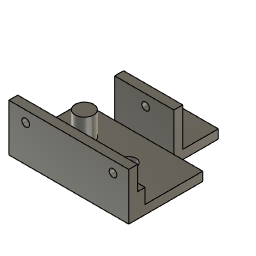
RoboCrab Top v3 (Autodesk Fusion 360 design; units mm, degrees)
Autodesk Fusion 360 part; units mm, degrees
sketch "Base" plane through (0, 0, 0) normal (0, 0, 1) x (1, 0, 0)
  line L0 (-9.4551, 20.4231) -> (10.5449, 20.4231)
  line L1 (20.2949, 5.4231) -> (20.2949, -19.5769)
  line L2 (20.2949, -19.5769) -> (-20.2051, -19.5769)
  line L3 (-20.2051, -19.5769) -> (-20.2051, 5.4231)
  line L4 (-20.2051, 5.4231) -> (-9.4551, 5.4231)
  line L5 (-9.4551, 5.4231) -> (-9.4551, 20.4231)
  line L6 (10.5449, 20.4231) -> (10.5449, 5.4231)
  line L7 (10.5449, 5.4231) -> (20.2949, 5.4231)
  dimension "d1" = 40
  dimension "d2" = 40.5
  dimension "d3" = 25
  dimension "d4" = 25
  dimension "d5" = 10.75
  dimension "d6" = 20
  constraint horizontal L0
  constraint vertical L1
  constraint horizontal L2
  constraint vertical L3
  constraint perpendicular L3 L4
  constraint perpendicular L0 L5
  constraint perpendicular L0 L6
  constraint perpendicular L1 L7
  measures "d1" distance of L0 L2
  measures "d2" distance of L1 L3
  measures "d3" distance of L2 L4
  measures "d4" distance of L2 L7
  measures "d5" distance of L3.end L4.end
  measures "d6" distance of L5 L6
extrude "Extrude1" add sketch "Base" along normal blind 3
sketch "Messurements" plane through (0, 0, 3) normal (0, 0, 1) x (-1, 0, 0)
  line L0 (-10.5449, -5.4231) -> (-10.5449, -20.4231)
  line L1 (-10.5449, -20.4231) -> (9.4551, -20.4231)
  line L2 (9.4551, -20.4231) -> (9.4551, -5.4231)
  line L3 (9.4551, -5.4231) -> (20.2051, -5.4231)
  line L4 (20.2051, -5.4231) -> (20.2051, 19.5769)
  line L5 (20.2051, 19.5769) -> (-20.2949, 19.5769)
  line L6 (-20.2949, 19.5769) -> (-20.2949, -5.4231)
  line L7 (-20.2949, -5.4231) -> (-10.5449, -5.4231)
  line L8 (20.2051, 14.0769) -> (-20.2949, 14.0769)
  line L9 (9.4551, -5.4231) -> (-10.5449, -5.4231)
  line L10 (9.4551, -8.4231) -> (-10.5449, -8.4231)
  circle A0 centre (-5.2949, 4.5769) radius 2.5
  circle A1 centre (9.6801, 4.5769) radius 3.125
  dimension "d9" = 5.5
  dimension "d10" = 3
  dimension "d11" = 5
  dimension "d12" = 6.25
  dimension "d13" = 15
  dimension "d14" = 10
  dimension "d15" = 10
  dimension "d16" = 10.525
  constraint coincident L4 L8.start
  constraint coincident L6 L8.end
  constraint perpendicular L6 L8
  constraint coincident L2.end L3.start
  constraint coincident L0.start L7.end
  constraint coincident L2 L10.start
  constraint coincident L0 L10.end
  constraint perpendicular L0 L10
  measures "d9" distance of L5 L8
  measures "d10" distance of L9 L10
  measures "d11" diameter of A0
  measures "d12" diameter of A1
  measures "d13" distance of L6 A0.centre
  measures "d14" distance of L9 A0.centre
  measures "d15" distance of L9 A1.centre
  measures "d16" distance of L4 A1.centre
extrude "Extrude2" cut sketch "Messurements" against normal blind 2 contours A0
extrude "Extrude3" add sketch "Messurements" along normal blind 8 contours A1
extrude "Extrude4" add sketch "Messurements" along normal blind 5 contours L4 L5 L6 L8
extrude "Extrude5" add sketch "Messurements" along normal blind 13 contours L0 L2 L9 L10
sketch "Other" plane through (0, 0, 8) normal (0, 0, 1) x (-1, 0, 0)
  line L0 (20.2051, 19.5769) -> (-20.2949, 19.5769)
  line L1 (-20.2949, 19.5769) -> (-20.2949, 14.0769)
  line L2 (-20.2949, 14.0769) -> (20.2051, 14.0769)
  line L3 (20.2051, 14.0769) -> (20.2051, 19.5769)
  line L4 (20.2051, 14.0769) -> (-20.2949, 14.0769)
  line L5 (-20.2949, 16.5769) -> (20.2051, 16.5769)
  dimension "d28" = 2.5
  constraint coincident L1 L5.start
  constraint coincident L3 L5.end
  constraint perpendicular L3 L5
  measures "d28" distance of L4 L5
extrude "Extrude6" add sketch "Other" along normal blind 8 contours L0 L1 L3 L5
sketch "Attachment2" plane through (0, -16.5769, 0) normal (0, 1, 0) x (-1, 0, 0)
  line L0 (-20.2949, 8) -> (20.2051, 8)
  line L1 (20.2051, 8) -> (20.2051, 16)
  line L2 (20.2051, 16) -> (-20.2949, 16)
  line L3 (-20.2949, 16) -> (-20.2949, 8)
  circle A0 centre (-14.9949, 12.3) radius 1.3
  circle A1 centre (14.5051, 12.3) radius 1.3
  dimension "d31" = 2.6
  dimension "d32" = 3.7
  dimension "d33" = 5.3
  dimension "d34" = 2.6
  dimension "d35" = 5.7
  dimension "d36" = 3.7
  measures "d31" diameter of A0
  measures "d32" distance of L2 A0.centre
  measures "d33" distance of L3 A0.centre
  measures "d34" diameter of A1
  measures "d35" distance of L1 A1.centre
  measures "d36" distance of L2 A1.centre
extrude "Extrude7" cut sketch "Attachment2" against normal through all contours A0
extrude "Extrude8" cut sketch "Attachment2" against normal through all contours A1
sketch "Attachment" plane through (0, 8.4231, 0) normal (0, 1, 0) x (-1, 0, 0)
  line L0 (-10.5449, 3) -> (9.4551, 3)
  line L1 (9.4551, 3) -> (9.4551, 16)
  line L2 (9.4551, 16) -> (-10.5449, 16)
  line L3 (-10.5449, 16) -> (-10.5449, 3)
  circle A0 centre (-0.9949, 12.3) radius 1.3
  dimension "d39" = 2.6
  dimension "d40" = 3.7
  dimension "d41" = 9.55
  measures "d39" diameter of A0
  measures "d40" distance of L2 A0.centre
  measures "d41" distance of L3 A0.centre
extrude "Extrude9" cut sketch "Attachment" against normal blind 4 contours A0
